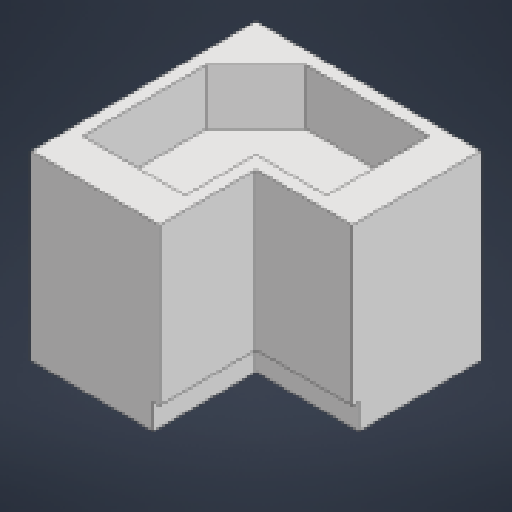
# Autodesk Inventor part: Mobile lavandino angolo
Saved by Autodesk Inventor 2024.2 (Build 282272000, 272)
## iProperties
Created: 2025-08-13
Part Number: Mobile lavandino angolo
Material: Generic
Document SubType Name: Modeling
Designer: Luca
Density: 1 g/cm^3
Appearance: Default
Author: Luca
Autodesk Inventor part; units mm, degrees
ref_plane "YZ Plane" through (0, 0, 0) normal (1, 0, 0) x (0, 1, 0)
ref_plane "XZ Plane" through (0, 0, 0) normal (0, 1, 0) x (-1, 0, 0)
ref_plane "XY Plane" through (0, 0, 0) normal (0, 0, 1) x (1, 0, 0)
sketch "Sketch1" plane through (0, 0, 0) normal (0, 1, 0) x (1, 0, 0)
  line L0 (300, 0) -> (-300, 0)
  line L1 (-300, 0) -> (-300, -600)
  line L2 (-300, -600) -> (300, -600)
  line L3 (300, -600) -> (300, 0)
  point P0 (0, 0)
  point P1 (0, 0)
  dimension "d0" = 600
  dimension "d1" = 600
  constraints: 8 end point, 2 parallel, 1 coincident, 1 horizontal, 1 midpoint, 1 perpendicular
  measures "d0" distance of L1.end L2.end
  measures "d1" distance of L0.end L1.end
extrude "Extrusion1" add sketch "Sketch1" along normal blind 850
sketch "Sketch2" plane through (-300, 0, 600) normal (0, 0, 1) x (-1, 0, 0)
  line L0 (-600, 0) -> (-600, -850) projected
  line L1 (-600, 0) -> (-570, 0)
  line L2 (-570, 0) -> (-570, -120)
  line L3 (-570, -120) -> (-600, -120)
  line L4 (-600, -120) -> (-600, 0)
  point P0 (-300, 0)
  dimension "d4" = 120
  dimension "d7" = 30
  constraints: 8 end point, 2 parallel, 1 horizontal, 1 perpendicular
  measures "d4" distance of L2.end L1.end
  measures "d7" distance between parallel lines of L0 L2
extrude "Extrusion2" cut sketch "Sketch2" against normal blind 30
move faces "Move3" translate (450, 0, 0) faces at (300, 323.3333, 190)
move faces "Move4" translate (0, 0, 450) faces at (240, 606.6667, 600)
sketch "Sketch3" plane through (270, 120, 570) normal (0, -1, 0) x (1, 0, 0)
  line L0 (-570, 480) -> (480, 480) projected
  line L1 (480, 480) -> (30, 480)
  line L2 (30, 480) -> (30, 30)
  line L3 (30, 30) -> (480, 30)
  line L4 (480, 30) -> (480, 480)
  line L5 (-570, 480) -> (-570, -570) projected
  line L6 (-570, -570) -> (480, -570) projected
  point P0 (-270, -570)
  point P1 (30, 480)
  dimension "d20" = 600
  dimension "d21" = 600
  constraints: 8 end point, 2 parallel, 1 horizontal, 1 perpendicular
  measures "d20" distance between parallel lines of L5 L2
  measures "d21" distance between parallel lines of L6 L3
extrude "Extrusion3" cut sketch "Sketch3" against normal through all
sketch "Sketch4" plane through (0, 850, 0) normal (0, 1, 0) x (1, 0, 0)
  line L0 (-240, -293.3452) -> (-6.6548, -60)
  line L1 (-6.6548, -60) -> (570, -60)
  line L2 (570, -60) -> (570, -540)
  line L3 (570, -540) -> (240, -540)
  line L4 (240, -540) -> (240, -870)
  line L5 (240, -870) -> (-240, -870)
  line L6 (-240, -870) -> (-240, -293.3452)
  line L7 (300, -600) -> (300, -1050) construction
  line L8 (240, -540) -> (300, -600) construction
  line L9 (-300, 0) -> (-300, -1050) projected
  point P0 (0, 0)
  point P1 (0, -870)
  dimension "d24" = 480
  dimension "d25" = 330
  dimension "d26" = 810
  dimension "d27" = 576.6548
  dimension "d28" = 330
  dimension "d29" = 300
  constraints: 16 end point, 9 perpendicular, 1 horizontal, 1 midpoint
  measures "d24" distance of L4.end L5.end
  measures "d25" distance of L0.start L0.end
  measures "d26" distance between parallel lines of L5 L1
  measures "d27" distance of L5.end L0.start
  measures "d28" distance of L2.end L3.end
  measures "d29" distance from line of point (0, -870) L9
extrude "Extrusion4" cut sketch "Sketch4" against normal blind 260
equation "\"d19\" = d16"
equation "\"d16\" = 450"
body "Solid1"
